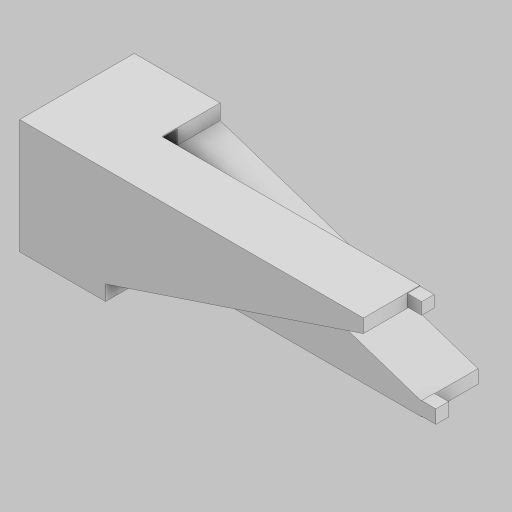
# Autodesk Inventor part: Hembra
Saved by Autodesk Inventor 2023 (Build 270158000, 158)
## iProperties
Created: 2026-02-22
Part Number: Hembra
Material: Genérico
Document SubType Name: Modeling
Designer: MARTIN MAESTRE
Density: 1 g/cm^3
Appearance: Valor por defecto
Author: MARTIN MAESTRE
Autodesk Inventor part; units mm, degrees
ref_plane "YZ Plane" through (0, 0, 0) normal (1, 0, 0) x (0, 1, 0)
ref_plane "XZ Plane" through (0, 0, 0) normal (0, 1, 0) x (-1, 0, 0)
ref_plane "XY Plane" through (0, 0, 0) normal (0, 0, 1) x (1, 0, 0)
sketch "Boceto1" plane through (0, 0, 0) normal (0, 0, 1) x (1, 0, 0)
  line L0 (0, 0) -> (120, 0)
  line L1 (0, 0) -> (0, 40)
  line L2 (0, 40) -> (120, 40)
  line L3 (120, 40) -> (120, 0)
  dimension "d0" = 120
  dimension "d1" = 40
  constraints: 8 end point, 2 perpendicular, 1 horizontal, 1 vertical
  measures "d0" distance of L0.start L0.end
  measures "d1" distance of L0.start L1.end
extrude "Extrusión1" add sketch "Boceto1" along normal blind 40
sketch "Boceto2" plane through (0, 0, 40) normal (0, 0, 1) x (1, 0, 0)
  line L0 (0, 0) -> (120, 0) construction
  line L1 (0, 0) -> (30, 0) construction
  line L2 (30, 0) -> (120, 0) construction
  line L3 (120, 0) -> (120, 35.3) construction
  line L4 (120, 0) -> (120, 40) construction
  line L5 (30, 0) -> (120, 0)
  line L6 (120, 35.3) -> (120, 0)
  line L7 (30, 0) -> (30, 5.3)
  line L8 (30, 5.3) -> (120, 35.3)
  line L9 (30, 0) -> (30, 0.3)
  line L10 (30, 0.3) -> (120, 0.3)
  line L11 (30, 0.3) -> (120, 0.3) construction
  dimension "d4" = 30
  dimension "d5" = 35.3
  dimension "d6" = 5.3
  dimension "d46" = 0.3
  dimension "d47" = 90
  dimension "d48" = 0
  constraints: 20 end point, 4 collinear, 3 point on line, 1 horizontal, 1 perpendicular, 1 vertical
  measures "d4" distance of L0.start L1.end
  measures "d5" distance of L0.end L3.end
  measures "d6" distance of L1.end L7.end
  measures "d46" distance of L1.end L9.end
  measures "d47" distance of L9.end L10.end
  measures "d48" distance between parallel lines of L10 L11
extrude "Extrusión2" cut sketch "Boceto2" against normal blind 20.3
sketch "Boceto3" plane through (0, 0, 0) normal (0, 0, -1) x (-1, 0, 0)
  line L0 (0, 0) -> (-120, 0) construction
  line L1 (0, 40) -> (0, 0) construction
  line L2 (0, 0) -> (0, 40) construction
  line L3 (0, 0) -> (40, 0) construction
  line L4 (0, 40) -> (-30, 40) construction
  line L5 (-120, 40) -> (0, 40) construction
  line L6 (-30, 40) -> (-30, 34.7)
  line L7 (0, 0) -> (-30, 0) construction
  line L8 (-120, 0) -> (-120, 40) projected
  line L9 (-30, 0) -> (-120, 0)
  line L10 (-120, 0) -> (-120, 4.7)
  line L11 (-120, 0) -> (-115.3, 0) construction
  line L12 (-120, 4.7) -> (-30, 34.7)
  line L13 (-120, 35.3) -> (-120, 40) projected
  line L14 (-120, 4.7) -> (-120, 40)
  line L15 (-120, 40) -> (-30, 40)
  dimension "d9" = 40
  dimension "d10" = 90
  dimension "d11" = 30
  dimension "d12" = 5.3
  dimension "d13" = 30
  dimension "d14" = 4.7
  dimension "d15" = 90
  constraints: 22 end point, 3 collinear, 3 horizontal, 2 perpendicular, 2 point on line, 2 vertical
  measures "d9" distance of L0.start L1.start
  measures "d10" angle of L3 L2
  measures "d11" distance of L1.start L4.end
  measures "d12" distance of L4.end L6.end
  measures "d13" distance of L0.start L7.end
  measures "d14" distance of L0.end L10.end
  measures "d15" angle of L11 L10
extrude "Extrusión3" cut sketch "Boceto3" against normal blind 20.3
sketch "Boceto4" plane through (120, 35.3, 40) normal (1, 0, 0) x (0, 0, -1)
  line L0 (0, 4.7) -> (0, -35.3) projected
  line L1 (0, 0.3857) -> (15.3, 0.3857)
  line L2 (0, 0.3857) -> (15.3, 0.3857) construction
  line L3 (15.3, 0.3857) -> (19.7, 0.3857)
  line L4 (19.7, 0.3857) -> (19.7, 4.4857)
  line L5 (19.7, 4.4857) -> (15.3, 4.4857)
  line L6 (15.3, 4.4857) -> (15.3, 0.3857)
  point P0 (40, -35.3)
  dimension "d18" = 15.3
  dimension "d19" = 0
  dimension "d20" = 4.4
  dimension "d21" = 4.1
  constraints: 12 end point, 2 horizontal, 2 parallel, 2 perpendicular, 1 collinear, 1 point on line
  measures "d18" distance of L1.start L1.end
  measures "d19" distance between parallel lines of L1 L2
  measures "d20" distance of L5.end L4.end
  measures "d21" distance of L4.end L3.end
extrude "Extrusión4" add sketch "Boceto4" along normal blind 5
sketch "Boceto6" plane through (30, 34.7, 0) normal (1, 0, 0) x (0, 0, -1)
  line L0 (0, 0) -> (-20.3, 0) projected
  line L1 (0, 0) -> (-15, 0)
  line L2 (-15, 0) -> (-20, 0)
  line L3 (-20, 0) -> (-20, 5)
  line L4 (-20, 5) -> (-15, 5)
  line L5 (-15, 5) -> (-15, 0)
  point P0 (0, -34.7)
  dimension "d28" = 15
  dimension "d29" = 5
  dimension "d30" = 5
  constraints: 10 end point, 2 parallel, 1 horizontal, 1 perpendicular, 1 point on line
  measures "d28" distance of L0.start L1.end
  measures "d29" distance of L3.end L4.end
  measures "d30" distance of L2.end L3.end
extrude "Extrusión6" cut sketch "Boceto6" against normal blind 5
sketch "Boceto7" plane through (30, 0, 40) normal (1, 0, 0) x (0, 0, -1)
  line L0 (20.3, 0) -> (0, 0) projected
  line L1 (0, 0) -> (15, 0)
  line L2 (15, 0) -> (20, 0)
  line L3 (20, 0) -> (20, 5)
  line L4 (20, 5) -> (15, 5)
  line L5 (15, 5) -> (15, 0)
  point P0 (40, 0)
  dimension "d33" = 15
  dimension "d34" = 5
  dimension "d35" = 5
  constraints: 10 end point, 2 parallel, 1 horizontal, 1 perpendicular, 1 point on line
  measures "d33" distance of L0.end L1.end
  measures "d34" distance of L4.end L3.end
  measures "d35" distance of L3.end L2.end
extrude "Extrusión7" cut sketch "Boceto7" against normal blind 5
sketch "Boceto8" plane through (120, 0, 19.7) normal (1, 0, 0) x (0, 0, -1)
  line L0 (0, 4.7) -> (0, 0) projected
  line L1 (0, 0) -> (0, 0)
  line L2 (0, 0) -> (0, 0) construction
  line L3 (0, 0) -> (0, 0.2)
  line L4 (19.7, 0) -> (-20.3, 0) projected
  line L5 (0, 0) -> (0.2, 0) construction
  line L6 (0, 0.2) -> (4.4, 0.2)
  line L7 (4.4, 0.2) -> (4.4, 4.9)
  line L8 (4.4, 4.9) -> (0, 4.9)
  line L9 (0, 4.9) -> (0, 0.2)
  dimension "d38" = 0
  dimension "d39" = 0
  dimension "d40" = 0.2
  dimension "d41" = 90
  dimension "d42" = 4.4
  dimension "d43" = 4.7
  constraints: 16 end point, 4 horizontal, 2 equal length, 2 parallel, 2 perpendicular
  measures "d38" distance of L0.end L1.end
  measures "d39" distance between parallel lines of L1 L2
  measures "d40" distance of L2.end L3.end
  measures "d41" angle of L5 L3
  measures "d42" distance of L8.end L7.end
  measures "d43" distance of L7.end L6.end
extrude "Extrusión8" add sketch "Boceto8" along normal blind 5
